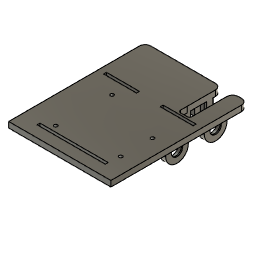
PlaqueAttache v11 (Autodesk Fusion 360 design; units mm, degrees)
Autodesk Fusion 360 part; units mm, degrees
sketch "Esquisse1" plane through (0, 0, 0) normal (0, 0, 1) x (1, 0, 0)
  line L0 (0, 0) -> (90, 0)
  line L1 (90, 0) -> (90, 83)
  line L2 (90, 83) -> (0, 83)
  line L3 (0, 83) -> (0, 0)
  dimension "d1" = 90
  dimension "d2" = 83
  constraint horizontal L0
  constraint vertical L1
  constraint horizontal L2
  constraint vertical L3
  constraint coincident L0.start L3.end
  measures "d1" distance of L1.end L2.end
  measures "d2" distance of L0.end L1.end
extrude "Extrusion1" add sketch "Esquisse1" along normal blind 5
sketch "Esquisse2" plane through (0, 0, 5) normal (0, 0, 1) x (-1, 0, 0)
  line L0 (0, -83) -> (0, 0)
  line L1 (0, 0) -> (-90, 0)
  line L2 (-90, 0) -> (-90, -83)
  line L3 (-90, -83) -> (0, -83)
  line L4 (-10, -10) -> (-82.576, -10)
  line L5 (-82.576, -10) -> (-82.576, -7.5)
  line L6 (-82.576, -7.5) -> (-10, -7.5)
  line L7 (-10, -7.5) -> (-10, -10)
  line L8 (-55.5, -80.5) -> (-84.5, -80.5)
  line L9 (-84.5, -80.5) -> (-84.5, -78)
  line L10 (-84.5, -78) -> (-55.5, -78)
  line L11 (-55.5, -78) -> (-55.5, -80.5)
  line L12 (-5.5, -80.5) -> (-34.5, -80.5)
  line L13 (-34.5, -80.5) -> (-34.5, -78)
  line L14 (-34.5, -78) -> (-5.5, -78)
  line L15 (-5.5, -78) -> (-5.5, -80.5)
  dimension "d5" = 2.5
  dimension "d6" = 2.5
  dimension "d8" = 2.5
  dimension "d9" = 29
  dimension "d10" = 5.5
  dimension "d11" = 5.5
  dimension "d12" = 29
  dimension "d13" = 2.5
  dimension "d14" = 2.5
  constraint horizontal L4
  constraint vertical L5
  constraint horizontal L6
  constraint vertical L7
  constraint horizontal L8
  constraint vertical L9
  constraint horizontal L10
  constraint vertical L11
  constraint horizontal L12
  constraint vertical L13
  constraint horizontal L14
  constraint vertical L15
  measures "d5" distance of L4.end L5.end
  measures "d6" distance of L8.end L9.end
  measures "d8" distance of L12.start L14.end
  measures "d9" distance of L8.start L8.end
  measures "d10" distance of L2 L9
  measures "d11" distance of L0 L15
  measures "d12" distance of L12.start L12.end
  measures "d13" distance of L3 L8
  measures "d14" distance of L3 L12
extrude "Extrusion2" cut sketch "Esquisse2" against normal blind 2.5 contours L8 L9 L10 L11 | L12 L13 L14 L15
sketch "Esquisse3" plane through (0, 0, 5) normal (0, 0, 1) x (-1, 0, 0)
  line L0 (-34.5, -80.5) -> (-34.5, -78)
  line L1 (-34.5, -78) -> (-5.5, -78)
  line L2 (-5.5, -78) -> (-5.5, -80.5)
  line L3 (-5.5, -80.5) -> (-34.5, -80.5)
  line L4 (-84.5, -80.5) -> (-84.5, -78)
  line L5 (-84.5, -78) -> (-55.5, -78)
  line L6 (-55.5, -78) -> (-55.5, -80.5)
  line L7 (-55.5, -80.5) -> (-84.5, -80.5)
  line L8 (0, -83) -> (0, 0)
  line L9 (0, 0) -> (-90, 0)
  line L10 (-90, 0) -> (-90, -83)
  line L11 (-90, -83) -> (0, -83)
  line L12 (-15, -12.5) -> (-75, -12.5)
  line L13 (-75, -12.5) -> (-75, -10)
  line L14 (-75, -10) -> (-15, -10)
  line L15 (-15, -10) -> (-15, -12.5)
  dimension "d17" = 2.5
  dimension "d18" = 10
  dimension "d19" = 60
  dimension "d20" = 15
  constraint horizontal L12
  constraint vertical L13
  constraint horizontal L14
  constraint vertical L15
  measures "d17" distance of L12.end L13.end
  measures "d18" distance of L9 L14
  measures "d19" distance of L12.start L12.end
  measures "d20" distance of L10 L13
extrude "Extrusion3" cut sketch "Esquisse3" against normal blind 3 contours L12 L13 L14 L15
sketch "Esquisse5" plane through (0, 83, 0) normal (0, 1, 0) x (-1, 0, 0)
  line L0 (-90, 0) -> (0, 0)
  line L1 (0, 0) -> (0, 5)
  line L2 (0, 5) -> (-90, 5)
  line L3 (-90, 5) -> (-90, 0)
  line L4 (-90, 5) -> (0, 5)
  line L5 (0, 5) -> (0, 0)
  line L6 (0, 0) -> (-90, 0)
  line L7 (-90, 0) -> (-90, 5)
  constraint horizontal L4
  constraint vertical L5
  constraint horizontal L6
  constraint vertical L7
  constraint coincident L0.end L1.start
  constraint coincident L2.end L3.start
extrude "Extrusion4" add sketch "Esquisse5" along normal blind 50
sketch "Esquisse4" plane through (0, 0, 0) normal (0, 0, -1) x (1, 0, 0)
  line L0 (0, 0) -> (0, -133)
  line L1 (90, -133) -> (90, 0)
  line L2 (90, 0) -> (0, 0)
  line L3 (64.5, -70.25) -> (25.5, -70.25)
  line L4 (33.5, -110.75) -> (33.5, -110.25)
  line L5 (53.5, -63.6293) -> (57.5, -63.6293)
  line L6 (25, -69.75) -> (65, -69.75)
  line L7 (65, -93.25) -> (67, -93.25)
  line L8 (65, -93.25) -> (64.5, -93.25)
  line L9 (53.5, -70.6293) -> (53.5, -63.6293)
  line L10 (23, -67.75) -> (67, -67.75)
  line L11 (53.5, -117.6433) -> (57.5, -117.6433)
  line L12 (65, -107.25) -> (67, -107.25)
  line L13 (25.5, -110.25) -> (64.5, -110.25)
  line L14 (53, -63.1293) -> (53, -69.75)
  line L15 (60, -69.75) -> (60, -61.1293)
  line L16 (60, -61.1293) -> (51, -61.1293)
  line L17 (58, -69.75) -> (58, -63.1293)
  line L18 (57.5, -70.25) -> (53.5, -70.6293)
  line L19 (65, -69.75) -> (65, -110.75)
  line L20 (51, -61.1293) -> (51, -69.75)
  line L21 (23, -112.75) -> (23, -67.75)
  line L22 (58, -110.75) -> (58, -118.1433)
  line L23 (28.5, -110.75) -> (28.5, -110.25)
  line L24 (65, -110.75) -> (25, -110.75)
  line L25 (33.5, -110.75) -> (33.5, -112.75)
  line L26 (28.5, -110.75) -> (28.5, -112.75)
  line L27 (65, -107.25) -> (64.5, -107.25)
  line L28 (60, -110.75) -> (60, -120.1433)
  line L29 (53, -118.1433) -> (53, -110.75)
  line L30 (67, -112.75) -> (23, -112.75)
  line L31 (53.5, -110.6433) -> (53.5, -117.6433)
  line L32 (60, -120.1433) -> (51, -120.1433)
  line L33 (58, -118.1433) -> (53, -118.1433)
  line L34 (57.5, -117.6433) -> (57.5, -110.25)
  line L35 (51, -120.1433) -> (51, -110.75)
  line L36 (57.5, -110.25) -> (53.5, -110.6433)
  line L37 (58, -63.1293) -> (53, -63.1293)
  line L38 (57.5, -63.6293) -> (57.5, -70.25)
  line L39 (67, -67.75) -> (67, -112.75)
  line L40 (25, -110.75) -> (25, -69.75)
  line L41 (64.5, -110.25) -> (64.5, -70.25)
  line L42 (25.5, -70.25) -> (25.5, -110.25)
  line L43 (65, -100.25) -> (67, -100.25)
  line L44 (0, -133) -> (90, -133)
  line L45 (51, -112.75) -> (46, -112.75)
  line L46 (46, -112.75) -> (46, -117.75)
  line L47 (46, -117.75) -> (51, -117.75)
  line L48 (51, -117.75) -> (51, -112.75)
  line L49 (48.5, -117.75) -> (48.5, -112.75)
  line L50 (51, -115.25) -> (46, -115.25)
  circle A0 centre (48.5, -115.25) radius 1
  line L51 (51, -67.75) -> (46, -67.75)
  line L52 (46, -67.75) -> (46, -62.75)
  line L53 (46, -62.75) -> (51, -62.75)
  line L54 (51, -62.75) -> (51, -67.75)
  line L55 (48.5, -62.75) -> (48.5, -67.75)
  line L56 (46, -65.25) -> (51, -65.25)
  circle A1 centre (48.5, -65.25) radius 1
  point P0 (64.5, -70.25)
  dimension "d23" = 40
  dimension "d24" = 39
  dimension "d25" = 7
  dimension "d26" = 7
  dimension "d27" = 4
  dimension "d28" = 4
  dimension "d29" = 7
  dimension "d30" = 7
  dimension "d31" = 0.5
  dimension "d32" = 0.5
  dimension "d33" = 0.5
  dimension "d34" = 0.5
  dimension "d35" = 0.5
  dimension "d36" = 0.5
  dimension "d37" = 0.5
  dimension "d38" = 0.5
  dimension "d39" = 0.5
  dimension "d40" = 0.5
  dimension "d41" = 5
  dimension "d42" = 3
  dimension "d43" = 14
  dimension "d44" = 3
  dimension "d45" = 2
  dimension "d46" = 2
  dimension "d47" = 2
  dimension "d48" = 2
  dimension "d49" = 2
  dimension "d50" = 2
  dimension "d51" = 2
  dimension "d52" = 2
  dimension "d53" = 2
  dimension "d54" = 2
  dimension "d55" = 7
  dimension "d58" = 23
  dimension "d61" = 100.25
  dimension "d113" = 5
  dimension "d114" = 5
  dimension "d115" = 2
  dimension "d116" = 5
  dimension "d117" = 5
  dimension "d118" = 2
  constraint coincident P0 L3.start
  constraint coincident L34.end L13
  constraint coincident L18.start L3
  constraint coincident L17.start L6
  constraint perpendicular L6 L17
  constraint perpendicular L17 L37
  constraint coincident L14.end L6
  constraint perpendicular L6 L14
  constraint coincident L22.start L24
  constraint perpendicular L22 L24
  constraint perpendicular L22 L33
  constraint coincident L29.end L24
  constraint perpendicular L29 L33
  constraint coincident L4.start L24
  constraint coincident L4.end L13
  constraint perpendicular L4 L13
  constraint coincident L23.start L24
  constraint coincident L23.end L13
  constraint perpendicular L13 L23
  constraint coincident L12.start L19
  constraint coincident L27.end L41
  constraint perpendicular L27 L41
  constraint coincident L7.start L19
  constraint coincident L8.end L41
  constraint perpendicular L8 L41
  constraint coincident L12.end L39
  constraint perpendicular L12 L39
  constraint coincident L7.end L39
  constraint perpendicular L7 L39
  constraint coincident L25.end L30
  constraint perpendicular L25 L30
  constraint coincident L26.end L30
  constraint perpendicular L26 L30
  constraint coincident L28.start L24
  constraint perpendicular L28 L30
  constraint perpendicular L22 L32
  constraint coincident L35.end L24
  constraint perpendicular L24 L35
  constraint coincident L15.start L6
  constraint perpendicular L6 L15
  constraint perpendicular L15 L16
  constraint coincident L20.end L6
  constraint perpendicular L6 L20
  constraint coincident L19 L43.start
  constraint coincident L39 L43.end
  constraint perpendicular L39 L43
  constraint horizontal L45
  constraint vertical L46
  constraint horizontal L47
  constraint vertical L48
  constraint coincident L35 L45.start
  constraint coincident L30 L45.start
  constraint midpoint L47 L49.start
  constraint midpoint L45 L49.end
  constraint midpoint L48 L50.start
  constraint midpoint L46 L50.end
  constraint midpoint L49 A0.centre
  constraint horizontal L51
  constraint vertical L52
  constraint horizontal L53
  constraint vertical L54
  constraint coincident L10 L51.start
  constraint coincident L20 L51.start
  constraint midpoint L53 L55.start
  constraint midpoint L51 L55.end
  constraint midpoint L52 L56.start
  constraint midpoint L54 L56.end
  constraint midpoint L55 A1.centre
  measures "d23" distance of L3.end L13.start
  measures "d24" distance of L13.end L13.start
  measures "d25" distance of L38 L41
  measures "d26" distance of L34 L41
  measures "d27" distance of L11.start L11.end
  measures "d28" distance of L5.start L5.end
  measures "d29" distance of L5.start L9.start
  measures "d30" distance of L11.start L31.start
  measures "d31" distance of L19 L41
  measures "d32" distance of L13 L24
  measures "d33" distance of L40 L42
  measures "d34" distance of L3 L6
  measures "d35" distance of L17 L38
  measures "d36" distance of L5 L37
  measures "d37" distance of L9 L14
  measures "d38" distance of L22 L34
  measures "d39" distance of L11 L33
  measures "d40" distance of L29 L31
  measures "d41" distance of L4 L23
  measures "d42" distance of L23 L42
  measures "d43" distance of L8 L27
  measures "d44" distance of L13 L27
  measures "d45" distance of L19 L39
  measures "d46" distance of L24 L30
  measures "d47" distance of L21 L40
  measures "d48" distance of L6 L10
  measures "d49" distance of L22 L28
  measures "d50" distance of L32 L33
  measures "d51" distance of L29 L35
  measures "d52" distance of L14 L20
  measures "d53" distance of L16 L37
  measures "d54" distance of L15 L17
  measures "d55" distance of L7 L43
  measures "d58" distance of L1 L39
  measures "d61" distance of L2 L43
  measures "d113" distance of L46.end L47.end
  measures "d114" distance of L45.end L46.end
  measures "d115" diameter of A0
  measures "d116" distance of L51.end L52.end
  measures "d117" distance of L52.end L53.end
  measures "d118" diameter of A1
extrude "Extrusion5" add sketch "Esquisse4" along normal blind 20 contours L6 L7 L10 L15 L19 L39 | L6 L10 L15 L17 | L12 L19 L24 L28 L30 L39 | L6 L10 L14 L20 | L10 L14 L15 L16 L17 L20 L37 L54 | L6 L10 L20 L21 L24 L26 L30 L40 L51 | L22 L24 L28 L30 | L10 L20 L51 L54 L55 L56 A1 | L22 L28 L29 L30 L32 L33 L35 L48 | L24 L25 L30 L35 L45 | L10 L51 L52 L55 L56 A1 | L20 L53 L54 L55 L56 A1 | L24 L29 L30 L35 | L30 L35 L45 L48 L49 L50 A0 | L30 L45 L46 L49 L50 A0 | L52 L53 L55 L56 A1 | L35 L47 L48 L49 L50 A0 | L46 L47 L49 L50 A0
sketch "Esquisse6" plane through (0, 0, 0) normal (0, 0, -1) x (1, 0, 0)
  line L0 (28.5, -110.75) -> (28.5, -112.75)
  line L1 (28.5, -112.75) -> (23, -112.75)
  line L2 (23, -112.75) -> (23, -67.75)
  line L3 (23, -67.75) -> (46, -67.75)
  line L4 (51, -62.75) -> (51, -61.1293)
  line L5 (51, -61.1293) -> (60, -61.1293)
  line L6 (60, -61.1293) -> (60, -67.75)
  line L7 (60, -67.75) -> (67, -67.75)
  line L8 (67, -67.75) -> (67, -93.25)
  line L9 (67, -93.25) -> (65, -93.25)
  line L10 (65, -93.25) -> (65, -69.75)
  line L11 (65, -69.75) -> (58, -69.75)
  line L12 (58, -69.75) -> (58, -63.1293)
  line L13 (58, -63.1293) -> (53, -63.1293)
  line L14 (53, -63.1293) -> (53, -69.75)
  line L15 (53, -69.75) -> (25, -69.75)
  line L16 (25, -69.75) -> (25, -110.75)
  line L17 (25, -110.75) -> (28.5, -110.75)
  line L18 (65, -110.75) -> (65, -107.25)
  line L19 (65, -107.25) -> (67, -107.25)
  line L20 (67, -107.25) -> (67, -112.75)
  line L21 (67, -112.75) -> (60, -112.75)
  line L22 (60, -112.75) -> (60, -120.1433)
  line L23 (60, -120.1433) -> (51, -120.1433)
  line L24 (51, -120.1433) -> (51, -117.75)
  line L25 (46, -112.75) -> (33.5, -112.75)
  line L26 (33.5, -112.75) -> (33.5, -110.75)
  line L27 (33.5, -110.75) -> (53, -110.75)
  line L28 (53, -110.75) -> (53, -118.1433)
  line L29 (53, -118.1433) -> (58, -118.1433)
  line L30 (58, -118.1433) -> (58, -110.75)
  line L31 (58, -110.75) -> (65, -110.75)
  line L32 (0, 0) -> (0, -133)
  line L33 (0, -133) -> (90, -133)
  line L34 (90, -133) -> (90, 0)
  line L35 (90, 0) -> (0, 0)
  line L36 (0, 0) -> (90, 0)
  line L37 (90, 0) -> (90, -83)
  line L38 (90, -83) -> (0, -83)
  line L39 (0, -83) -> (0, 0)
  line L40 (67, -83) -> (67, -112.75)
  line L41 (60, -112.75) -> (60, -120.1433)
  line L42 (23, -112.75) -> (46, -112.75)
  line L43 (67, -112.75) -> (60, -112.75)
  line L44 (23, -112.75) -> (23, -83)
  line L45 (51, -117.75) -> (46, -117.75)
  line L46 (46, -117.75) -> (46, -112.75)
  line L47 (46, -67.75) -> (46, -62.75)
  line L48 (46, -62.75) -> (51, -62.75)
  dimension "d64" = 83
  constraint horizontal L36
  constraint vertical L37
  constraint horizontal L38
  constraint vertical L39
  constraint coincident L34 L37.end
  constraint coincident L32.start L35.end
  constraint coincident L38 L40.start
  constraint coincident L8 L40.start
  constraint coincident L20.end L21.start
  constraint coincident L21.end L22.start
  constraint coincident L22.end L23.start
  constraint coincident L1.end L2.start
  constraint coincident L25.start L42.end
  constraint coincident L38 L44.end
  constraint coincident L2 L44.end
  measures "d64" distance of L34.end L37.end
extrude "Extrusion6" cut sketch "Esquisse6" against normal blind 5 contours L1 L2 L8 L20 L21 L22 L23 L24 L25 L32 L33 L34 L38 L40 L41 L42 L43 L44 L45 L46
sketch "Esquisse7" plane through (0, 83, 0) normal (0, 1, 0) x (-1, 0, 0)
  line L0 (-90, 0) -> (-67, 0)
  line L1 (-67, 0) -> (-67, 5)
  line L2 (-67, 5) -> (-90, 5)
  line L3 (-90, 5) -> (-90, 0)
  line L4 (-67, 0) -> (-72, 0)
  line L5 (-72, 0) -> (-72, 5)
  line L6 (-72, 5) -> (-67, 5)
  line L7 (-67, 5) -> (-67, 0)
  line L8 (-72, 5) -> (-75, 5)
  line L9 (-75, 5) -> (-75, 0)
  line L10 (-75, 0) -> (-72, 0)
  line L11 (-72, 0) -> (-72, 5)
  line L12 (-75, 0) -> (-77, 0)
  line L13 (-77, 0) -> (-77, 5)
  line L14 (-77, 5) -> (-75, 5)
  line L15 (-75, 5) -> (-75, 0)
  line L16 (-77, 5) -> (-82, 5)
  line L17 (-82, 5) -> (-82, 0)
  line L18 (-82, 0) -> (-77, 0)
  line L19 (-77, 0) -> (-77, 5)
  dimension "d67" = 5
  dimension "d68" = 3
  dimension "d69" = 2
  dimension "d70" = 5
  constraint horizontal L4
  constraint vertical L5
  constraint horizontal L6
  constraint vertical L7
  constraint coincident L2 L5.end
  constraint coincident L0.end L1.start
  constraint horizontal L8
  constraint vertical L9
  constraint horizontal L10
  constraint vertical L11
  constraint coincident L0 L9.end
  constraint horizontal L12
  constraint vertical L13
  constraint horizontal L14
  constraint vertical L15
  constraint coincident L2 L13.end
  constraint horizontal L16
  constraint vertical L17
  constraint horizontal L18
  constraint vertical L19
  constraint coincident L0 L17.end
  measures "d67" distance of L5.end L1.end
  measures "d68" distance of L5.end L8.end
  measures "d69" distance of L13.end L8.end
  measures "d70" distance of L13.end L16.end
extrude "Extrusion7" add sketch "Esquisse7" along normal blind 25 contours L0 L2 L13 L16 L17 L18 L19
sketch "Esquisse8" plane through (0, 0, 0) normal (0, 0, -1) x (1, 0, 0)
  line L0 (0, -83) -> (23, -83)
  line L1 (23, -83) -> (23, -67.75)
  line L2 (23, -67.75) -> (46, -67.75)
  line L3 (51, -62.75) -> (51, -61.1293)
  line L4 (51, -61.1293) -> (60, -61.1293)
  line L5 (60, -61.1293) -> (60, -67.75)
  line L6 (60, -67.75) -> (67, -67.75)
  line L7 (67, -67.75) -> (67, -83)
  line L8 (67, -83) -> (77, -83)
  line L9 (77, -83) -> (77, -108)
  line L10 (77, -108) -> (82, -108)
  line L11 (82, -108) -> (82, -83)
  line L12 (82, -83) -> (90, -83)
  line L13 (90, -83) -> (90, 0)
  line L14 (90, 0) -> (0, 0)
  line L15 (0, 0) -> (0, -83)
  line L16 (82, -100.25) -> (77, -100.25)
  line L17 (77, -100.25) -> (77, 0)
  line L18 (77, 0) -> (82, 0)
  line L19 (82, 0) -> (82, -100.25)
  line L20 (82, -106.75) -> (77, -106.75)
  line L21 (77, -106.75) -> (77, -93.75)
  line L22 (77, -93.75) -> (82, -93.75)
  line L23 (82, -93.75) -> (82, -106.75)
  line L24 (46, -67.75) -> (46, -62.75)
  line L25 (46, -62.75) -> (51, -62.75)
  dimension "d73" = 100.25
  dimension "d74" = 13
  dimension "d75" = 6.5
  constraint horizontal L16
  constraint vertical L17
  constraint horizontal L18
  constraint vertical L19
  constraint coincident L14 L17.end
  constraint coincident L11 L16.start
  constraint horizontal L20
  constraint vertical L21
  constraint horizontal L22
  constraint vertical L23
  constraint coincident L9 L21.end
  constraint coincident L17 L21.end
  constraint coincident L11 L20.start
  measures "d73" distance of L16.start L18.end
  measures "d74" distance of L20.end L21.end
  measures "d75" distance of L16 L20
extrude "Extrusion8" add sketch "Esquisse8" along normal blind 1 contours L9 L11 L16 L17 L19 L21 L22 L23 | L9 L11 L16 L20 L21 L23
sketch "Esquisse9" plane through (77, 0, 0) normal (-1, 0, 0) x (0, -1, 0)
  line L0 (-83, 0) -> (-83, 5)
  line L1 (-83, 5) -> (-108, 5)
  line L2 (-108, 5) -> (-108, 0)
  line L3 (-108, 0) -> (-106.75, 0)
  line L4 (-106.75, 0) -> (-93.75, 0)
  line L5 (-93.75, 0) -> (-83, 0)
  line L6 (-106.75, 0) -> (-93.75, 0)
  line L7 (-106.75, 0) -> (-100.25, 0)
  line L8 (-100.25, 0) -> (-100.25, -9)
  circle A0 centre (-100.25, -9) radius 7
  circle A1 centre (-100.25, -9) radius 10
  line L9 (-100.25, -9) -> (-110.25, -9)
  line L10 (-100.25, -9) -> (-90.25, -9)
  line L11 (-110.25, -9) -> (-110.25, 0)
  line L12 (-110.25, 0) -> (-106.75, 0)
  line L13 (-90.25, -9) -> (-90.25, 0)
  line L14 (-90.25, 0) -> (-93.75, 0)
  dimension "d78" = 6.5
  dimension "d79" = 14
  dimension "d80" = 9
  dimension "d81" = 20
  constraint coincident L3.end L4.start
  constraint coincident L4.end L5.start
  constraint coincident L4 L7.end
  constraint perpendicular L7 L8
  constraint coincident L8.end A0.centre
  constraint concentric A0 A1
  constraint coincident A1 L9.end
  constraint perpendicular L8 L9
  constraint coincident A1 L10.end
  constraint perpendicular L8 L10
  constraint coincident L3 L11.end
  constraint tangent A1 L11
  constraint coincident L5 L13.end
  constraint tangent A1 L13
  measures "d78" distance of L3.end L7.end
  measures "d79" diameter of A0
  measures "d80" distance of L7.end L8.end
  measures "d81" diameter of A1
extrude "Extrusion9" add sketch "Esquisse9" against normal blind 5 contours L4 L5 L6 A1 L13 L14 | L4 L6 L8 A0 A1 L10 | A0 A1 L9 L10 | L3 L4 L6 L7 A1 L11 L12 | L4 L6 L7 A1 | L4 L6 L7 L8 A0 A1 L9
sketch "Esquisse10" plane through (82, 0, 0) normal (1, 0, 0) x (0, 1, 0)
  circle A0 centre (100.25, -9) radius 7
  line L0 (90.25, 0) -> (90.25, -9)
  arc A1 (90.25, -9) -> (110.25, -9) centre (100.25, -9) ccw
  line L1 (110.25, -9) -> (110.25, 0)
  line L2 (108, 0) -> (108, 5)
  line L3 (108, 5) -> (83, 5)
  line L4 (83, 5) -> (83, 0)
  line L5 (83, 0) -> (90.25, 0)
  circle A2 centre (100.25, -9) radius 6.5
  circle A3 centre (100.25, -9) radius 7.5
  circle A4 centre (100.25, -9) radius 5
  line L6 (110.25, 0) -> (108, 0)
  dimension "d84" = 15
  dimension "d85" = 13
  dimension "d86" = 10
  constraint concentric A0 A2
  constraint concentric A0 A3
  constraint concentric A2 A4
  measures "d84" diameter of A3
  measures "d85" diameter of A2
  measures "d86" diameter of A4
extrude "Extrusion10" add sketch "Esquisse10" against normal blind 1 contours A0 | A2
sketch "Esquisse11" plane through (0, 83, 0) normal (0, 1, 0) x (-1, 0, 0)
  line L0 (-23, 0) -> (0, 0)
  line L1 (0, 0) -> (0, 5)
  line L2 (0, 5) -> (-23, 5)
  line L3 (-23, 5) -> (-23, 0)
  line L4 (0, 5) -> (-8, 5)
  line L5 (-8, 5) -> (-8, 0)
  line L6 (-8, 0) -> (0, 0)
  line L7 (0, 0) -> (0, 5)
  line L8 (-8, 5) -> (-13, 5)
  line L9 (-13, 5) -> (-13, 0)
  line L10 (-13, 0) -> (-8, 0)
  line L11 (-8, 0) -> (-8, 5)
  dimension "d89" = 8
  dimension "d90" = 5
  constraint horizontal L4
  constraint vertical L5
  constraint horizontal L6
  constraint vertical L7
  constraint coincident L0 L5.end
  constraint coincident L1.end L2.start
  constraint horizontal L8
  constraint vertical L9
  constraint horizontal L10
  constraint vertical L11
  constraint coincident L0 L9.end
  measures "d89" distance of L1.end L4.end
  measures "d90" distance of L4.end L8.end
extrude "Extrusion11" add sketch "Esquisse11" along normal blind 25 contours L0 L2 L5 L8 L9 L10 L11
sketch "Esquisse12" plane through (8, 0, 0) normal (-1, 0, 0) x (0, -1, 0)
  line L0 (-83, 0) -> (-83, 5)
  line L1 (-83, 5) -> (-108, 5)
  line L2 (-108, 5) -> (-108, 0)
  line L3 (-108, 0) -> (-83, 0)
  line L4 (-108, 0) -> (-110.25, 0)
  line L5 (-110.25, 0) -> (-110.25, 5)
  line L6 (-110.25, 5) -> (-108, 5)
  line L7 (-108, 5) -> (-108, 0)
  line L8 (-110.25, 0) -> (-90.25, 0)
  line L9 (-90.25, 0) -> (-90.25, 5)
  line L10 (-90.25, 5) -> (-110.25, 5)
  line L11 (-110.25, 5) -> (-110.25, 0)
  line L12 (-90.25, 0) -> (-100.25, 0)
  line L13 (-100.25, 0) -> (-100.25, -9)
  circle A0 centre (-100.25, -9) radius 7
  circle A1 centre (-100.25, -9) radius 10
  line L14 (-100.25, -9) -> (-110.25, -9)
  line L15 (-100.25, -9) -> (-90.25, -9)
  line L16 (-90.25, -9) -> (-90.25, 0)
  line L17 (-110.25, -9) -> (-110.25, 0)
  dimension "d94" = 20
  dimension "d95" = 14
  dimension "d96" = 9
  dimension "d97" = 20
  dimension "d186" = 7.25
  constraint horizontal L4
  constraint vertical L5
  constraint horizontal L6
  constraint vertical L7
  constraint coincident L1 L5.end
  constraint coincident L2.end L3.start
  constraint horizontal L8
  constraint vertical L9
  constraint horizontal L10
  constraint vertical L11
  constraint coincident L1 L9.end
  constraint midpoint L8 L12.end
  constraint perpendicular L3 L13
  constraint coincident L13.end A0.centre
  constraint concentric A0 A1
  constraint coincident A1 L14.end
  constraint perpendicular L13 L14
  constraint coincident A1 L15.end
  constraint perpendicular L13 L15
  measures "d94" distance of L4.end L8.end
  measures "d95" diameter of A0
  measures "d96" distance of L12.end L13.end
  measures "d97" diameter of A1
  measures "d186" distance of L0 L9
extrude "Extrusion12" add sketch "Esquisse12" against normal blind 5 contours L3 L8 L12 A1 L16 | L3 L8 L12 L13 A0 A1 L15 | L3 L8 L12 A1 | A0 A1 L14 L15 | L3 L8 L13 A0 A1 L14 | L3 L4 L8 A1 L17
sketch "Esquisse13" plane through (8, 0, 0) normal (-1, 0, 0) x (0, -1, 0)
  line L0 (-83, 0) -> (-83, 5)
  line L1 (-83, 5) -> (-108, 5)
  line L2 (-108, 5) -> (-108, 0)
  line L3 (-110.25, 0) -> (-110.25, -9)
  arc A0 (-110.25, -9) -> (-90.25, -9) centre (-100.25, -9) ccw
  line L4 (-90.25, -9) -> (-90.25, 0)
  line L5 (-90.25, 0) -> (-83, 0)
  circle A1 centre (-100.25, -9) radius 7.5
  circle A2 centre (-100.25, -9) radius 5
  line L6 (-108, 0) -> (-110.25, 0)
  dimension "d100" = 15
  dimension "d102" = 10
  constraint concentric A1 A2
  measures "d100" diameter of A1
  measures "d102" diameter of A2
extrude "Extrusion13" add sketch "Esquisse13" against normal blind 1 contours A1
sketch "Esquisse14" plane through (0, 0, 0) normal (0, 0, -1) x (1, 0, 0)
  line L0 (8, -90.25) -> (13, -90.25)
  line L1 (13, -90.25) -> (13, -83)
  line L2 (13, -83) -> (23, -83)
  line L3 (23, -83) -> (23, -67.75)
  line L4 (23, -67.75) -> (46, -67.75)
  line L5 (46, -67.75) -> (46, -62.75)
  line L6 (46, -62.75) -> (51, -62.75)
  line L7 (51, -62.75) -> (51, -61.1293)
  line L8 (51, -61.1293) -> (60, -61.1293)
  line L9 (60, -61.1293) -> (60, -67.75)
  line L10 (60, -67.75) -> (67, -67.75)
  line L11 (67, -67.75) -> (67, -83)
  line L12 (67, -83) -> (77, -83)
  line L13 (77, -83) -> (77, -90.25)
  line L14 (77, -90.25) -> (82, -90.25)
  line L15 (82, -90.25) -> (82, -83)
  line L16 (82, -83) -> (90, -83)
  line L17 (90, -83) -> (90, 0)
  line L18 (90, 0) -> (0, 0)
  line L19 (0, 0) -> (0, -83)
  line L20 (0, -83) -> (8, -83)
  line L21 (8, -83) -> (8, -90.25)
  line L22 (82, -90.25) -> (77, -90.25)
  line L23 (77, -90.25) -> (77, -58.75)
  line L24 (77, -58.75) -> (82, -58.75)
  line L25 (82, -58.75) -> (82, -90.25)
  line L26 (77, -58.75) -> (82, -58.75)
  line L27 (82, -58.75) -> (82, -73.75)
  line L28 (82, -73.75) -> (77, -73.75)
  line L29 (77, -73.75) -> (77, -58.75)
  line L30 (13, -90.25) -> (8, -90.25)
  line L31 (8, -90.25) -> (8, -58.75)
  line L32 (8, -58.75) -> (13, -58.75)
  line L33 (13, -58.75) -> (13, -90.25)
  line L34 (13, -58.75) -> (8, -58.75)
  line L35 (8, -58.75) -> (8, -73.75)
  line L36 (8, -73.75) -> (13, -73.75)
  line L37 (13, -73.75) -> (13, -58.75)
  dimension "d119" = 31.5
  dimension "d120" = 5
  dimension "d121" = 15
  dimension "d122" = 5
  dimension "d123" = 31.5
  dimension "d124" = 15
  constraint horizontal L22
  constraint vertical L23
  constraint horizontal L24
  constraint vertical L25
  constraint coincident L14.end L15.start
  constraint horizontal L26
  constraint vertical L27
  constraint horizontal L28
  constraint vertical L29
  constraint coincident L25 L27.end
  constraint horizontal L30
  constraint vertical L31
  constraint horizontal L32
  constraint vertical L33
  constraint coincident L0.end L1.start
  constraint horizontal L34
  constraint vertical L35
  constraint horizontal L36
  constraint vertical L37
  constraint coincident L31 L35.end
  measures "d119" distance of L13.end L23.end
  measures "d120" distance of L23.end L24.end
  measures "d121" distance of L24 L28
  measures "d122" distance of L31.end L32.end
  measures "d123" distance of L0.start L31.end
  measures "d124" distance of L32 L36
extrude "Extrusion14" add sketch "Esquisse14" along normal blind 1 contours L31 L32 L33 L34 L35 L36 L37 | L23 L24 L25 L26 L27 L28 L29
sketch "Esquisse15" plane through (82, 0, 0) normal (1, 0, 0) x (0, 1, 0)
  line L0 (73.75, 0) -> (58.75, 0)
  line L1 (58.75, 0) -> (58.75, -1)
  line L2 (58.75, -1) -> (73.75, -1)
  line L3 (73.75, -1) -> (73.75, 0)
  line L4 (73.75, 0) -> (58.75, 0)
  line L5 (66.25, 0) -> (66.25, -9)
  circle A0 centre (66.25, -9) radius 7
  circle A1 centre (66.25, -9) radius 10
  line L6 (66.25, -9) -> (56.25, -9)
  line L7 (66.25, -9) -> (76.25, -9)
  line L8 (76.25, -9) -> (76.25, 0)
  line L9 (56.25, -9) -> (56.25, 0)
  line L10 (56.25, 0) -> (76.25, 0)
  dimension "d127" = 14
  dimension "d128" = 9
  dimension "d129" = 20
  constraint coincident L0.start L3.end
  constraint coincident L0.end L1.start
  constraint midpoint L4 L5.start
  constraint perpendicular L0 L5
  constraint coincident L5.end A0.centre
  constraint concentric A0 A1
  constraint coincident A1 L6.end
  constraint perpendicular L5 L6
  constraint coincident A1 L7.end
  constraint parallel L6 L7
  constraint tangent A1 L8
  constraint tangent A1 L9
  constraint perpendicular L8 L10
  measures "d127" diameter of A0
  measures "d128" distance of L5.start L5.end
  measures "d129" diameter of A1
extrude "Extrusion15" add sketch "Esquisse15" against normal blind 5 contours L0 L2 L3 L4 A1 L10 | L2 L3 A1 L8 L10 | L0 L2 L4 L5 A1 L10 | L0 L2 L4 L5 A1 L10 | L2 L5 A0 A1 L7 | L0 L1 L2 L4 A1 L10 | A0 A1 L6 L7 | L2 L5 A0 A1 L6 | L1 L2 A1 L9 L10
sketch "Esquisse16" plane through (82, 0, 0) normal (1, 0, 0) x (0, 1, 0)
  line L0 (76.25, 0) -> (56.25, 0)
  circle A0 centre (66.25, -9) radius 6.5
  circle A1 centre (66.25, -9) radius 7.5
  circle A2 centre (66.25, -9) radius 5
  circle A3 centre (66.25, -9) radius 7
  line L1 (56.25, 0) -> (56.25, -9)
  arc A4 (56.25, -9) -> (76.25, -9) centre (66.25, -9) ccw
  line L2 (76.25, -9) -> (76.25, 0)
  dimension "d132" = 15
  dimension "d133" = 13
  dimension "d134" = 10
  dimension "d190" = 10
  constraint concentric A0 A1
  constraint concentric A0 A2
  measures "d132" diameter of A1
  measures "d133" diameter of A0
  measures "d134" diameter of A2
  measures "d190" distance of A0.centre A4.end
extrude "Extrusion16" add sketch "Esquisse16" against normal blind 1 contours A0 | A1 | A3
sketch "Esquisse17" plane through (8, 0, 0) normal (-1, 0, 0) x (0, -1, 0)
  line L0 (-58.75, 0) -> (-73.75, 0)
  line L1 (-73.75, 0) -> (-73.75, -1)
  line L2 (-73.75, -1) -> (-58.75, -1)
  line L3 (-58.75, -1) -> (-58.75, 0)
  line L4 (-58.75, 0) -> (-73.75, 0)
  line L5 (-58.75, 0) -> (-66.25, 0)
  line L6 (-66.25, 0) -> (-66.25, -9)
  circle A0 centre (-66.25, -9) radius 7
  circle A1 centre (-66.25, -9) radius 10
  line L7 (-66.25, -9) -> (-56.25, -9)
  line L8 (-66.25, -9) -> (-76.25, -9)
  line L9 (-56.25, -9) -> (-56.25, 0)
  line L10 (-76.25, -9) -> (-76.25, 0)
  line L11 (-76.25, 0) -> (-56.25, 0)
  dimension "d137" = 14
  dimension "d138" = 9
  dimension "d139" = 20
  constraint coincident L0.start L3.end
  constraint coincident L0.end L1.start
  constraint midpoint L4 L5.end
  constraint perpendicular L2 L6
  constraint coincident L6.end A0.centre
  constraint concentric A0 A1
  constraint coincident A1 L7.end
  constraint perpendicular L6 L7
  constraint coincident A1 L8.end
  constraint parallel L7 L8
  constraint tangent A1 L9
  constraint tangent A1 L10
  constraint perpendicular L9 L11
  measures "d137" diameter of A0
  measures "d138" distance of L5.end L6.end
  measures "d139" diameter of A1
extrude "Extrusion17" add sketch "Esquisse17" against normal blind 5 contours L0 L2 L3 L4 L5 A1 L11 | L2 L3 A1 L9 L11 | L0 L2 L4 L5 L6 A1 L11 | L0 L4 L5 A1 L11 | L0 L2 L4 L6 A1 L11 | L2 L6 A0 A1 L7 | L0 L1 L2 L4 A1 L11 | A0 A1 L7 L8 | L2 L6 A0 A1 L8 | L1 L2 A1 L10 L11
sketch "Esquisse18" plane through (8, 0, 0) normal (-1, 0, 0) x (0, -1, 0)
  line L0 (-56.25, 0) -> (-76.25, 0)
  arc A0 (-76.25, -9) -> (-56.25, -9) centre (-66.25, -9) ccw
  circle A1 centre (-66.25, -9) radius 6.5
  circle A2 centre (-66.25, -9) radius 7.5
  circle A3 centre (-66.25, -9) radius 5
  line L1 (-76.25, 0) -> (-76.25, -9)
  circle A4 centre (-66.25, -9) radius 7
  line L2 (-56.25, -9) -> (-56.25, 0)
  dimension "d142" = 15
  dimension "d143" = 13
  dimension "d144" = 10
  dimension "d191" = 10
  dimension "d192" = 10
  constraint concentric A1 A3
  measures "d142" diameter of A2
  measures "d143" diameter of A1
  measures "d144" diameter of A3
  measures "d191" distance of A0.centre L1
  measures "d192" distance of A0.centre L1
extrude "Extrusion18" add sketch "Esquisse18" against normal blind 1 contours A1 | A2 | A4
sketch "Esquisse19" plane through (0, 0, 5) normal (0, 0, 1) x (-1, 0, 0)
  line L0 (-23, -83) -> (-13, -83)
  line L1 (-13, -83) -> (-13, -108)
  line L2 (-13, -108) -> (-8, -108)
  line L3 (-8, -108) -> (-8, -83)
  line L4 (-8, -83) -> (0, -83)
  line L5 (0, -83) -> (0, 0)
  line L6 (0, 0) -> (-90, 0)
  line L7 (-90, 0) -> (-90, -83)
  line L8 (-90, -83) -> (-82, -83)
  line L9 (-82, -83) -> (-82, -108)
  line L10 (-82, -108) -> (-77, -108)
  line L11 (-77, -108) -> (-77, -83)
  line L12 (-77, -83) -> (-67, -83)
  line L13 (-67, -83) -> (-67, -112.75)
  line L14 (-67, -112.75) -> (-60, -112.75)
  line L15 (-60, -112.75) -> (-60, -120.1433)
  line L16 (-60, -120.1433) -> (-51, -120.1433)
  line L17 (-51, -120.1433) -> (-51, -117.75)
  line L18 (-51, -117.75) -> (-46, -117.75)
  line L19 (-46, -117.75) -> (-46, -112.75)
  line L20 (-46, -112.75) -> (-23, -112.75)
  line L21 (-23, -112.75) -> (-23, -83)
  line L22 (-75, -12.5) -> (-75, -10)
  line L23 (-75, -10) -> (-15, -10)
  line L24 (-15, -10) -> (-15, -12.5)
  line L25 (-15, -12.5) -> (-75, -12.5)
  line L26 (-34.5, -80.5) -> (-34.5, -78)
  line L27 (-34.5, -78) -> (-5.5, -78)
  line L28 (-5.5, -78) -> (-5.5, -80.5)
  line L29 (-5.5, -80.5) -> (-34.5, -80.5)
  line L30 (-84.5, -80.5) -> (-84.5, -78)
  line L31 (-84.5, -78) -> (-55.5, -78)
  line L32 (-55.5, -78) -> (-55.5, -80.5)
  line L33 (-55.5, -80.5) -> (-84.5, -80.5)
  line L34 (-10, -68.34) -> (-78.58, -68.34)
  line L35 (-78.58, -68.34) -> (-78.58, -15)
  line L36 (-78.58, -15) -> (-10, -15)
  line L37 (-10, -15) -> (-10, -68.34)
  circle A0 centre (-76.04, -22.62) radius 1.5
  circle A1 centre (-76.04, -50.56) radius 1.5
  circle A2 centre (-25.24, -65.8) radius 1.5
  circle A3 centre (-23.97, -17.54) radius 1.5
  dimension "d147" = 68.58
  dimension "d148" = 53.34
  dimension "d149" = 10
  dimension "d150" = 15
  dimension "d151" = 3
  dimension "d152" = 3
  dimension "d153" = 3
  dimension "d154" = 3
  dimension "d155" = 66.04
  dimension "d156" = 45.72
  dimension "d157" = 66.04
  dimension "d158" = 17.78
  dimension "d159" = 50.8
  dimension "d160" = 13.97
  dimension "d161" = 50.8
  dimension "d162" = 15.24
  constraint horizontal L34
  constraint vertical L35
  constraint horizontal L36
  constraint vertical L37
  measures "d147" distance of L34.start L34.end
  measures "d148" distance of L34.start L36.end
  measures "d149" distance of L5 L37
  measures "d150" distance of L6 L36
  measures "d151" diameter of A0
  measures "d152" diameter of A2
  measures "d153" diameter of A3
  measures "d154" diameter of A1
  measures "d155" distance of L37 A0.centre
  measures "d156" distance of L34 A0.centre
  measures "d157" distance of L37 A1.centre
  measures "d158" distance of L34 A1.centre
  measures "d159" distance of L34 A3.centre
  measures "d160" distance of L37 A3.centre
  measures "d161" distance of L36 A2.centre
  measures "d162" distance of L37 A2.centre
extrude "Extrusion19" cut sketch "Esquisse19" against normal blind 5 contours A0 | A1 | A2 | A3
sketch "Esquisse20" plane through (0, 0, 0) normal (0, 0, -1) x (1, 0, 0)
  line L0 (82, -56.25) -> (82, -76.25)
  line L1 (8, -76.25) -> (8, -56.25)
  line L2 (13, -56.25) -> (13, -76.25)
  line L3 (82, -83) -> (90, -83)
  line L4 (90, -83) -> (90, 0)
  line L5 (90, 0) -> (0, 0)
  line L6 (0, 0) -> (0, -83)
  line L7 (0, -83) -> (8, -83)
  line L8 (13, -90.25) -> (13, -83)
  line L9 (13, -83) -> (23, -83)
  line L10 (23, -83) -> (23, -67.75)
  line L11 (23, -67.75) -> (46, -67.75)
  line L12 (46, -67.75) -> (46, -62.75)
  line L13 (46, -62.75) -> (51, -62.75)
  line L14 (51, -62.75) -> (51, -61.1293)
  line L15 (51, -61.1293) -> (60, -61.1293)
  line L16 (60, -61.1293) -> (60, -67.75)
  line L17 (60, -67.75) -> (67, -67.75)
  line L18 (67, -67.75) -> (67, -83)
  line L19 (67, -83) -> (77, -83)
  line L20 (77, -83) -> (77, -90.25)
  circle A0 centre (23.97, -17.54) radius 1.5
  circle A1 centre (25.24, -65.8) radius 1.5
  circle A2 centre (76.04, -22.62) radius 1.5
  line L21 (67, -67.75) -> (62, -67.75)
  line L22 (62, -67.75) -> (62, -52.75)
  line L23 (62, -52.75) -> (67, -52.75)
  line L24 (67, -52.75) -> (67, -67.75)
  line L25 (23, -67.75) -> (28, -67.75)
  line L26 (28, -67.75) -> (28, -52.75)
  line L27 (28, -52.75) -> (23, -52.75)
  line L28 (23, -52.75) -> (23, -67.75)
  circle A3 centre (25.24, -65.8) radius 1.5
  line L29 (8, -83) -> (8, -90.25)
  line L30 (82, -90.25) -> (82, -83)
  line L31 (8, -90.25) -> (13, -90.25)
  line L32 (77, -90.25) -> (82, -90.25)
  line L33 (77, -56.25) -> (82, -56.25)
  line L34 (82, -76.25) -> (77, -76.25)
  line L35 (77, -76.25) -> (77, -56.25)
  line L36 (13, -76.25) -> (8, -76.25)
  line L37 (8, -56.25) -> (13, -56.25)
  circle A4 centre (76.04, -50.56) radius 1.5
  dimension "d175" = 5
  dimension "d176" = 15
  dimension "d177" = 15
  dimension "d178" = 5
  dimension "d179" = 3
  constraint horizontal L21
  constraint vertical L22
  constraint horizontal L23
  constraint vertical L24
  constraint coincident L17.end L18.start
  constraint horizontal L25
  constraint vertical L26
  constraint horizontal L27
  constraint vertical L28
  constraint coincident L10.end L11.start
  constraint concentric A1 A3
  measures "d175" distance of L26.end L27.end
  measures "d176" distance of L25.end L26.end
  measures "d177" distance of L21.end L22.end
  measures "d178" distance of L22.end L23.end
  measures "d179" diameter of A3
extrude "Extrusion20" add sketch "Esquisse20" along normal blind 20 contours L17 L21 L22 L23 L24 | L11 L25 L26 L27 L28
sketch "Esquisse21" plane through (0, 83, 0) normal (0, 1, 0) x (-1, 0, 0)
  line L0 (-82, 0) -> (-82, 5)
  line L1 (-82, 5) -> (-90, 5)
  line L2 (-90, 5) -> (-90, 0)
  line L3 (-90, 0) -> (-82, 0)
  line L4 (-90, 0) -> (0, 0)
  line L5 (0, 0) -> (0, 5)
  line L6 (0, 5) -> (-90, 5)
  line L7 (-90, 5) -> (-90, 0)
  dimension "d182" = 90
  dimension "d183" = 5
  constraint horizontal L4
  constraint vertical L5
  constraint horizontal L6
  constraint vertical L7
  constraint coincident L2.end L3.start
  measures "d182" distance of L5.end L1.end
  measures "d183" distance of L4.end L5.end
extrude "Extrusion21" add sketch "Esquisse21" along normal blind 37.143
sketch "Esquisse23" plane through (0, 0, 0) normal (0, 0, -1) x (1, 0, 0)
  line L0 (90, -120.143) -> (90, 0)
  line L1 (90, 0) -> (0, 0)
  line L2 (0, 0) -> (0, -120.143)
  line L3 (0, -120.143) -> (51, -120.143)
  line L4 (51, -120.143) -> (51, -117.75)
  line L5 (51, -117.75) -> (46, -117.75)
  line L6 (46, -117.75) -> (46, -112.75)
  line L7 (46, -112.75) -> (33.5, -112.75)
  line L8 (33.5, -112.75) -> (33.5, -110.75)
  line L9 (33.5, -110.75) -> (53, -110.75)
  line L10 (53, -110.75) -> (53, -118.1433)
  line L11 (53, -118.1433) -> (58, -118.1433)
  line L12 (58, -118.1433) -> (58, -110.75)
  line L13 (58, -110.75) -> (65, -110.75)
  line L14 (65, -110.75) -> (65, -107.25)
  line L15 (65, -107.25) -> (67, -107.25)
  line L16 (67, -107.25) -> (67, -112.75)
  line L17 (67, -112.75) -> (60, -112.75)
  line L18 (60, -112.75) -> (60, -120.143)
  line L19 (60, -120.143) -> (90, -120.143)
  line L20 (8, -90.25) -> (13, -90.25)
  line L21 (13, -90.25) -> (13, -110.25)
  line L22 (13, -110.25) -> (8, -110.25)
  line L23 (8, -110.25) -> (8, -90.25)
  line L24 (82, -90.25) -> (82, -110.25)
  line L25 (82, -110.25) -> (77, -110.25)
  line L26 (77, -110.25) -> (77, -106.75)
  line L27 (77, -106.75) -> (77, -93.75)
  line L28 (77, -93.75) -> (77, -90.25)
  line L29 (77, -90.25) -> (82, -90.25)
  line L30 (67, -52.75) -> (67, -93.25)
  line L31 (67, -93.25) -> (65, -93.25)
  line L32 (65, -93.25) -> (65, -69.75)
  line L33 (65, -69.75) -> (58, -69.75)
  line L34 (58, -69.75) -> (58, -63.1293)
  line L35 (58, -63.1293) -> (53, -63.1293)
  line L36 (53, -63.1293) -> (53, -69.75)
  line L37 (53, -69.75) -> (25, -69.75)
  line L38 (25, -69.75) -> (25, -110.75)
  line L39 (25, -110.75) -> (28.5, -110.75)
  line L40 (28.5, -110.75) -> (28.5, -112.75)
  line L41 (28.5, -112.75) -> (23, -112.75)
  line L42 (23, -112.75) -> (23, -52.75)
  line L43 (23, -52.75) -> (28, -52.75)
  line L44 (28, -52.75) -> (28, -67.75)
  line L45 (28, -67.75) -> (46, -67.75)
  line L46 (46, -67.75) -> (46, -62.75)
  line L47 (46, -62.75) -> (51, -62.75)
  line L48 (51, -62.75) -> (51, -61.1293)
  line L49 (51, -61.1293) -> (60, -61.1293)
  line L50 (60, -61.1293) -> (60, -67.75)
  line L51 (60, -67.75) -> (62, -67.75)
  line L52 (62, -67.75) -> (62, -52.75)
  line L53 (62, -52.75) -> (67, -52.75)
  line L54 (8, -76.25) -> (8, -56.25)
  line L55 (8, -56.25) -> (13, -56.25)
  line L56 (13, -56.25) -> (13, -76.25)
  line L57 (13, -76.25) -> (8, -76.25)
  line L58 (82, -56.25) -> (82, -76.25)
  line L59 (82, -76.25) -> (77, -76.25)
  line L60 (77, -76.25) -> (77, -56.25)
  line L61 (77, -56.25) -> (82, -56.25)
  circle A0 centre (23.97, -17.54) radius 1.5
  circle A1 centre (76.04, -50.56) radius 1.5
  circle A2 centre (76.04, -22.62) radius 1.5
  line L62 (77, -56.25) -> (67, -56.25)
  line L63 (67, -56.25) -> (67, -76.25)
  line L64 (67, -76.25) -> (77, -76.25)
  line L65 (77, -76.25) -> (77, -56.25)
  line L66 (13, -56.25) -> (23, -56.25)
  line L67 (23, -56.25) -> (23, -76.25)
  line L68 (23, -76.25) -> (13, -76.25)
  line L69 (13, -76.25) -> (13, -56.25)
  line L70 (67, -56.25) -> (69.5, -56.25)
  line L71 (69.5, -56.25) -> (69.5, -76.25)
  line L72 (69.5, -76.25) -> (67, -76.25)
  line L73 (67, -76.25) -> (67, -56.25)
  line L74 (23, -56.25) -> (20.5, -56.25)
  line L75 (20.5, -56.25) -> (20.5, -76.25)
  line L76 (20.5, -76.25) -> (23, -76.25)
  line L77 (23, -76.25) -> (23, -56.25)
  line L78 (23, -76.25) -> (20.5, -76.25)
  line L79 (20.5, -76.25) -> (20.5, -110.25)
  line L80 (20.5, -110.25) -> (23, -110.25)
  line L81 (23, -110.25) -> (23, -76.25)
  dimension "d193" = 20
  dimension "d194" = 20
  dimension "d195" = 2.5
  dimension "d196" = 2.5
  dimension "d197" = 2.5
  dimension "d198" = 34
  constraint horizontal L62
  constraint vertical L63
  constraint horizontal L64
  constraint vertical L65
  constraint coincident L30 L63.end
  constraint coincident L60.end L61.start
  constraint horizontal L66
  constraint vertical L67
  constraint horizontal L68
  constraint vertical L69
  constraint coincident L42 L67.end
  constraint coincident L55.end L56.start
  constraint horizontal L70
  constraint vertical L71
  constraint horizontal L72
  constraint vertical L73
  constraint coincident L64 L71.end
  constraint horizontal L74
  constraint vertical L75
  constraint horizontal L76
  constraint vertical L77
  constraint coincident L68 L75.end
  constraint horizontal L78
  constraint vertical L79
  constraint horizontal L80
  constraint vertical L81
  measures "d193" distance of L60.end L59.end
  measures "d194" distance of L55.end L56.end
  measures "d195" distance of L71 L73
  measures "d196" distance of L75 L77
  measures "d197" distance of L79.end L80.end
  measures "d198" distance of L75.end L79.end
extrude "Extrusion23" add sketch "Esquisse23" along normal blind 20 contours L30 L62 L63 L64 L70 L71 L72 L73 | L42 L66 L67 L68 L74 L75 L76 L77 L78 | L42 L68 L76 L78 L79 L80 L81
sketch "Esquisse24" plane through (0, 0, 0) normal (0, 0, -1) x (1, 0, 0)
  line L0 (69.5, -76.25) -> (67, -76.25)
  line L1 (67, -76.25) -> (67, -93.25)
  line L2 (67, -93.25) -> (65, -93.25)
  line L3 (65, -93.25) -> (65, -69.75)
  line L4 (65, -69.75) -> (58, -69.75)
  line L5 (58, -69.75) -> (58, -63.1293)
  line L6 (58, -63.1293) -> (53, -63.1293)
  line L7 (53, -63.1293) -> (53, -69.75)
  line L8 (53, -69.75) -> (25, -69.75)
  line L9 (25, -69.75) -> (25, -110.75)
  line L10 (25, -110.75) -> (28.5, -110.75)
  line L11 (28.5, -110.75) -> (28.5, -112.75)
  line L12 (28.5, -112.75) -> (23, -112.75)
  line L13 (23, -112.75) -> (23, -110.25)
  line L14 (23, -110.25) -> (20.5, -110.25)
  line L15 (20.5, -110.25) -> (20.5, -56.25)
  line L16 (20.5, -56.25) -> (23, -56.25)
  line L17 (23, -56.25) -> (23, -52.75)
  line L18 (23, -52.75) -> (28, -52.75)
  line L19 (28, -52.75) -> (28, -67.75)
  line L20 (28, -67.75) -> (46, -67.75)
  line L21 (46, -67.75) -> (46, -62.75)
  line L22 (46, -62.75) -> (51, -62.75)
  line L23 (51, -62.75) -> (51, -61.1293)
  line L24 (51, -61.1293) -> (60, -61.1293)
  line L25 (60, -61.1293) -> (60, -67.75)
  line L26 (60, -67.75) -> (62, -67.75)
  line L27 (62, -67.75) -> (62, -52.75)
  line L28 (62, -52.75) -> (67, -52.75)
  line L29 (67, -52.75) -> (67, -56.25)
  line L30 (67, -56.25) -> (69.5, -56.25)
  line L31 (69.5, -56.25) -> (69.5, -76.25)
  circle A0 centre (76.04, -22.62) radius 1.5
  circle A1 centre (76.04, -50.56) radius 1.5
  circle A2 centre (23.97, -17.54) radius 1.5
  line L32 (82, -56.25) -> (82, -76.25)
  line L33 (82, -76.25) -> (77, -76.25)
  line L34 (77, -76.25) -> (77, -56.25)
  line L35 (77, -56.25) -> (82, -56.25)
  line L36 (8, -76.25) -> (8, -56.25)
  line L37 (8, -56.25) -> (13, -56.25)
  line L38 (13, -56.25) -> (13, -76.25)
  line L39 (13, -76.25) -> (8, -76.25)
  line L40 (82, -90.25) -> (82, -110.25)
  line L41 (82, -110.25) -> (77, -110.25)
  line L42 (77, -110.25) -> (77, -106.75)
  line L43 (77, -106.75) -> (77, -93.75)
  line L44 (77, -93.75) -> (77, -90.25)
  line L45 (77, -90.25) -> (82, -90.25)
  line L46 (8, -90.25) -> (13, -90.25)
  line L47 (13, -90.25) -> (13, -110.25)
  line L48 (13, -110.25) -> (8, -110.25)
  line L49 (8, -110.25) -> (8, -90.25)
  line L50 (90, -120.143) -> (90, 0)
  line L51 (90, 0) -> (0, 0)
  line L52 (0, 0) -> (0, -120.143)
  line L53 (0, -120.143) -> (51, -120.143)
  line L54 (51, -120.143) -> (51, -117.75)
  line L55 (51, -117.75) -> (46, -117.75)
  line L56 (46, -117.75) -> (46, -112.75)
  line L57 (46, -112.75) -> (33.5, -112.75)
  line L58 (33.5, -112.75) -> (33.5, -110.75)
  line L59 (33.5, -110.75) -> (53, -110.75)
  line L60 (53, -110.75) -> (53, -118.1433)
  line L61 (53, -118.1433) -> (58, -118.1433)
  line L62 (58, -118.1433) -> (58, -110.75)
  line L63 (58, -110.75) -> (65, -110.75)
  line L64 (65, -110.75) -> (65, -107.25)
  line L65 (65, -107.25) -> (67, -107.25)
  line L66 (67, -107.25) -> (67, -112.75)
  line L67 (67, -112.75) -> (60, -112.75)
  line L68 (60, -112.75) -> (60, -120.143)
  line L69 (60, -120.143) -> (90, -120.143)
  line L70 (77, -90.25) -> (67, -90.25)
  line L71 (67, -90.25) -> (67, -120.143)
  line L72 (67, -120.143) -> (77, -120.143)
  line L73 (77, -120.143) -> (77, -90.25)
  line L74 (77, -90.25) -> (67, -90.25)
  line L75 (67, -90.25) -> (67, -76.25)
  line L76 (67, -76.25) -> (77, -76.25)
  line L77 (77, -76.25) -> (77, -90.25)
  line L78 (77, -90.25) -> (67, -90.25)
  line L79 (67, -90.25) -> (67, -82.25)
  line L80 (67, -82.25) -> (77, -82.25)
  line L81 (77, -82.25) -> (77, -90.25)
  dimension "d201" = 10
  dimension "d202" = 8
  constraint horizontal L70
  constraint vertical L71
  constraint horizontal L72
  constraint vertical L73
  constraint coincident L69 L71.end
  constraint coincident L44.end L45.start
  constraint horizontal L74
  constraint vertical L75
  constraint horizontal L76
  constraint vertical L77
  constraint coincident L0.end L1.start
  constraint horizontal L78
  constraint vertical L79
  constraint horizontal L80
  constraint vertical L81
  constraint coincident L1 L79.end
  measures "d201" distance of L71.end L72.end
  measures "d202" distance of L70.end L79.end
extrude "Extrusion24" cut sketch "Esquisse24" against normal blind 5 contours L1 L70 L74 L75 L77 L78 L79 L80 L81 | L1 L42 L43 L44 L66 L69 L70 L71 L72 L73 L74 L78
fillet "Congé10" radius 2 2 edges at (77, 82.25, 2.5) (67, 82.25, 2.5)
fillet "Congé11" radius 5 4 edges at (90, 120.143, 2.5) (77, 120.143, 2.5) (67, 120.143, 2.5) (0, 120.143, 2.5)
fillet "Congé12" radius 5 3 edges at (79.5, 110.25, 0) (79.5, 90.25, 0) (79.5, 76.25, 0)
fillet "Congé13" radius 5 4 edges at (10.5, 110.25, 0) (10.5, 76.25, 0) (10.5, 90.25, 0) (10.5, 56.25, 0)
fillet "Congé14" radius 2.5 4 edges at (8, 66.25, 0) (8, 100.25, 0) (82, 100.25, 0) (82, 68.75, 0)
fillet "Congé15" radius 2 1 edges at (80.75, 56.25, 0)
